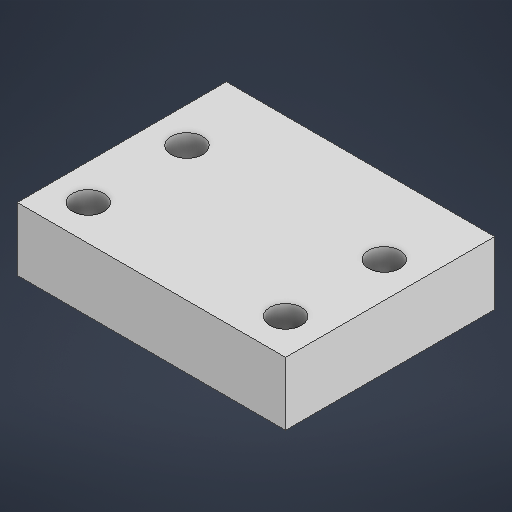
# Autodesk Inventor part: bottomMotorMount
Saved by Autodesk Inventor 2026.2 (Build 302298000, 298)
## iProperties
Created: 2026-09-23
Part Number: bottomMotorMount
Material: Generic
Document SubType Name: Modeling
Designer: Brian Wang
Density: 1 g/cm^3
Appearance: Default
Author: Brian Wang
Autodesk Inventor part; units mm, degrees
ref_plane "YZ Plane" through (0, 0, 0) normal (1, 0, 0) x (0, 1, 0)
ref_plane "XZ Plane" through (0, 0, 0) normal (0, 1, 0) x (-1, 0, 0)
ref_plane "XY Plane" through (0, 0, 0) normal (0, 0, 1) x (1, 0, 0)
sketch "Sketch1" plane through (0, 0, 0) normal (0, 1, 0) x (-1, 0, 0)
  line L0 (7.4046, 11.4154) -> (-60.5954, 11.4154)
  line L1 (-60.5954, 11.4154) -> (-60.5954, -41.5846)
  line L2 (-60.5954, -41.5846) -> (7.4046, -41.5846)
  line L3 (7.4046, -41.5846) -> (7.4046, 11.4154)
  point P0 (0, 0)
  dimension "d0" = 68
  dimension "d1" = 53
  constraints: 8 end point, 2 parallel, 1 horizontal, 1 perpendicular
  measures "d0" distance of L2.end L1.end
  measures "d1" distance of L1.end L0.end
extrude "Extrusion1" add sketch "Sketch1" along normal blind 16
sketch "Sketch2" plane through (0, 16, 0) normal (0, 1, 0) x (1, 0, 0)
  circle A0 centre (1.5954, -2.4154) radius 4
  circle A1 centre (1.5954, 22.5846) radius 4
  circle A2 centre (51.5954, 22.5846) radius 4
  circle A3 centre (51.5954, -2.4154) radius 4
  line L0 (-7.4046, 41.5846) -> (-7.4046, -11.4154) projected
  line L1 (-7.4046, -11.4154) -> (60.5954, -11.4154) projected
  point P0 (0, 0)
  dimension "d4" = 8
  dimension "d5" = 8
  dimension "d6" = 8
  dimension "d7" = 8
  dimension "d8" = 50
  dimension "d9" = 25
  dimension "d10" = 9
  dimension "d11" = 9
  constraints: 4 centre point, 2 horizontal alignment, 2 vertical alignment
  measures "d4" diameter of A0
  measures "d5" diameter of A1
  measures "d6" diameter of A2
  measures "d7" diameter of A3
  measures "d8" distance of A3.centre A0.centre
  measures "d9" distance of A1.centre A0.centre
  measures "d10" distance from line of L0 A0.centre
  measures "d11" distance from line of L1 A0.centre
extrude "Extrusion2" cut sketch "Sketch2" against normal blind 14
sketch "Sketch3" plane through (1.5954, 2, 2.4154) normal (0, 1, 0) x (1, 0, 0)
  circle A0 centre (0, 0) radius 4 projected
  circle A1 centre (0, 0) radius 1.7
  circle A2 centre (0, 25) radius 4 projected
  circle A3 centre (0, 25) radius 1.7
  circle A4 centre (50, 25) radius 4 projected
  circle A5 centre (50, 25) radius 1.7
  circle A6 centre (50, 0) radius 4 projected
  circle A7 centre (50, 0) radius 1.7
  point P0 (-1.5954, 2.4154)
  dimension "d14" = 3.4
  dimension "d15" = 3.4
  dimension "d16" = 3.4
  dimension "d17" = 3.4
  constraints: 4 centre point, 4 coincident
  measures "d14" diameter of A1
  measures "d15" diameter of A3
  measures "d16" diameter of A5
  measures "d17" diameter of A7
extrude "Extrusion3" cut sketch "Sketch3" against normal through all contours A1 | A3 | A5 | A7
body "Solid1"
